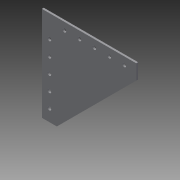
# Autodesk Inventor part: HolonomicCornerBracket
Saved by Autodesk Inventor 2013 SP2 (Build 170200200, 200)
## iProperties
Created: 2015-01-07
Part Number: HolonomicCornerBracket
Material: Generic
Document SubType Name: Sheet Metal
Designer: darkb_000
Density: 1 g/cm^3
Sheet Metal Rule: Default
Author: darkb_000
BendRadius: 0.125 in
BendReliefWidth: 0.125 in
BendReliefDepth: 0.063 in
CornerReliefSize: 0.500 in
MinimumRemnant: 0.250 in
TransitionRadius: 0.125 in
JacobiRadiusSize: 0.125 in
GapSize: 0.125 in
d0: 0.500 in
Thickness: 0.125 in
d1: 0.125 in
d2: 5.000 in
d3: 5.000 in
d4: 1.000 in
d5: 0.125 in
d6: 0.00 deg
d7: 0.125 in
d8: 0.063 in
d9: 0.250 in
d10: 0.125 in
d11: 4.000 in
d12: 90.00 deg
d13: 0.125 in
d14: 0.500 in
d15: 0.125 in
d16: 0.125 in
d17: 0.125 in
d18: 0.00 deg
d19: 1.250 in
d20: 1.250 in
d21: 1.250 in
d22: 1.250 in
d23: 0.125 in
d24: 0.00 deg
Autodesk Inventor part; units mm, degrees
ref_plane "YZ Plane" through (0, 0, 0) normal (1, 0, 0) x (0, 1, 0)
ref_plane "XZ Plane" through (0, 0, 0) normal (0, 1, 0) x (-1, 0, 0)
ref_plane "XY Plane" through (0, 0, 0) normal (0, 0, 1) x (1, 0, 0)
sketch "Sketch1" plane through (0, 0, 0) normal (0, 0, 1) x (1, 0, 0)
  line L0 (-313.0099, -160.8742) -> (-169.3258, -17.1901)
  line L1 (342.9, 12.7) -> (-342.9, 12.7)
  line L2 (-342.9, -12.7) -> (-342.9, -673.1)
  line L3 (-241.1678, -89.0322) -> (-250.1481, -80.0519)
  line L4 (-250.1481, -80.0519) -> (-157.3962, 12.7)
  line L5 (-157.3962, 12.7) -> (-342.9, 12.7)
  line L6 (-157.3962, 12.7) -> (-342.9, -172.8038)
  line L7 (-342.9, -172.8038) -> (-342.9, 12.7)
  circle A0 centre (-203.2, 0) radius 3.175
  circle A1 centre (-228.6, 0) radius 3.175
  circle A2 centre (-254, 0) radius 3.175
  circle A3 centre (-279.4, 0) radius 3.175
  circle A4 centre (-304.8, 0) radius 3.175
  circle A5 centre (-330.2, -25.4) radius 3.175
  circle A6 centre (-330.2, -50.8) radius 3.175
  circle A7 centre (-330.2, -76.2) radius 3.175
  circle A8 centre (-330.2, -101.6) radius 3.175
  circle A9 centre (-330.2, -127) radius 3.175
  line L8 (342.9, -12.7) -> (-342.9, -12.7)
  line L9 (-317.5, -12.7) -> (-317.5, -673.1)
  line L10 (-182.7962, -12.7) -> (-182.7962, 12.7)
  line L11 (-317.5, -147.4038) -> (-342.9, -147.4038)
  point P0 (0, 0)
  dimension "d0" = 12.7
  measures "d0" distance of L3.start L3.end
extrude "Plate1" add sketch "Sketch1" along normal blind 3.175 contours L10 L8 L7 L1 | L4 L6 L9 L8 | L9 L11 L2 L8
sketch "Sketch2" plane through (0, 0, 3.175) normal (0, 0, 1) x (1, 0, 0)
  circle A0 centre (-330.2, -127) radius 3.175 projected
  circle A1 centre (-203.2, 0) radius 3.175 projected
  line L0 (-182.7962, -12.7) -> (-317.5, -147.4038) projected
  line L1 (-342.9, 12.7) -> (-182.7962, 12.7) projected
  line L2 (-342.9, -147.4038) -> (-342.9, 12.7) projected
  line L3 (-317.5, -147.4038) -> (-342.9, -147.4038) projected
  line L4 (-317.5, -114.3) -> (-342.9, -114.3)
  line L5 (-215.9, 12.7) -> (-342.9, 12.7)
  line L6 (-342.9, 12.7) -> (-342.9, -114.3)
  line L7 (-342.9, -114.3) -> (-317.5, -114.3)
  line L8 (-317.5, -114.3) -> (-215.9, -12.7)
  line L9 (-215.9, -114.3) -> (-215.9, -45.8038)
  line L10 (-215.9, -12.7) -> (-215.9, 12.7)
  line L11 (-342.9, -114.3) -> (-317.5, -114.3)
  line L12 (-284.3962, -114.3) -> (-215.9, -114.3)
  line L13 (-215.9, 12.7) -> (-182.7962, 12.7)
  line L14 (-182.7962, 12.7) -> (-182.7962, -12.7)
  line L15 (-182.7962, -12.7) -> (-317.5, -147.4038)
  line L16 (-317.5, -147.4038) -> (-342.9, -147.4038)
  line L17 (-342.9, -147.4038) -> (-342.9, -114.3)
  point P0 (0, 0)
  dimension "d2" = 127
  dimension "d3" = 127
  dimension "d4" = 25.4
  constraints: 28 end point, 6 perpendicular, 5 parallel, 4 collinear, 3 point on line, 2 horizontal
  measures "d2" distance of L5.end L5.start
  measures "d3" distance of L5.start L9.start
  measures "d4" distance of L4.start L4.end
extrude "Cut1" cut sketch "Sketch2" against normal blind 3.175 contours L0 L3 L2 L4 L8 L10 L1 L14
sketch "Sketch3" plane through (-315.2549, -116.5451, -3.175) normal (0.7071068, -0.7071068, 0) x (0.7071068, 0.7071068, 0)
  line L0 (143.6841, 0) -> (0, 0)
  line L1 (0, 0) -> (0, -95.25)
  line L2 (0, -95.25) -> (143.6841, -95.25)
  line L3 (143.6841, -95.25) -> (143.6841, 0)
  constraints: 6 end point, 1 horizontal, 1 perpendicular, 1 vertical
edge flange "Flange1" height 101.6 angle 90 thickness 3.175 bend radius 3.175 thickness toward (0.7071068, -0.7071068, 0) relief tear relief width 3.175 relief depth 1.5875 edges at (-266.7, -63.5, 0) wall of the first edge with corners at (-213.6549, -14.9451, -3.175) (-315.2549, -116.5451, -3.175) (-315.2549, -116.5451, -98.425) (-213.6549, -14.9451, -98.425)
bend "Bend1"
corner "Corner1"
sketch "Sketch4" plane through (-313.0099, -118.7901, -3.175) normal (0.7071068, -0.7071068, 0) x (-0.7071068, -0.7071068, 0)
  line L0 (0, 95.25) -> (0, 0) projected
  line L1 (-174.6104, 73.025) -> (-37.9584, 73.025) projected
  line L2 (-176.1344, 73.025) -> (32.4504, 73.025) projected
  circle A0 centre (-71.842, 34.925) radius 10.8585 projected
  line L3 (0, 73.025) -> (-143.6841, 73.025)
  line L4 (-143.6841, 73.025) -> (-143.6841, 95.25)
  line L5 (-143.6841, 95.25) -> (0, 95.25)
  line L6 (0, 95.25) -> (0, 73.025)
  circle A1 centre (-71.842, 34.925) radius 10.8585
  point P0 (-305.3287, -3.175)
  constraints: 8 end point, 2 parallel, 2 point on line, 1 centre point, 1 coincident, 1 concentric, 1 horizontal, 1 perpendicular
extrude "Cut2" cut sketch "Sketch4" against normal blind 3.175
sketch "Sketch5" plane through (-211.4099, -17.1901, -3.175) normal (0.7071068, -0.7071068, 0) x (-0.7071068, -0.7071068, 0)
  line L0 (0, 73.025) -> (31.75, 73.025)
  line L1 (31.75, 73.025) -> (31.75, 41.275)
  line L2 (31.75, 41.275) -> (0, 41.275)
  line L3 (0, 41.275) -> (0, 73.025)
  line L4 (143.6841, 73.025) -> (111.9341, 73.025)
  line L5 (111.9341, 73.025) -> (111.9341, 41.275)
  line L6 (111.9341, 41.275) -> (143.6841, 41.275)
  line L7 (143.6841, 41.275) -> (143.6841, 73.025)
  line L8 (31.75, 73.025) -> (0, 41.275)
  line L9 (111.9341, 73.025) -> (143.6841, 41.275)
  point P0 (-161.6446, -3.175)
  dimension "d19" = 31.75
  dimension "d20" = 31.75
  dimension "d21" = 31.75
  dimension "d22" = 31.75
  constraints: 20 end point, 4 parallel, 2 horizontal, 2 perpendicular
  measures "d19" distance of L1.end L2.end
  measures "d20" distance of L0.end L1.end
  measures "d21" distance of L6.end L5.end
  measures "d22" distance of L5.end L4.end
extrude "Cut3" cut sketch "Sketch5" against normal blind 3.175 contours L0 L8 L3 | L7 L9 L4
equation "\"d5\" = Thickness"
equation "\"d17\" = Thickness"
equation "\"d23\" = Thickness"
equation "\"d7\" = BendReliefWidth"
equation "\"d8\" = BendReliefDepth"
equation "\"d9\" = MinimumRemnant"
equation "\"d10\" = BendRadius"
equation "\"d13\" = BendRadius"
equation "\"d14\" = CornerReliefSize"
equation "\"d15\" = GapSize"
equation "\"d16\" = JacobiRadiusSize"
equation "\"BendRadius\" = Thickness"
equation "\"BendReliefWidth\" = Thickness"
equation "\"BendReliefDepth\" = 0.5 * Thickness"
equation "\"CornerReliefSize\" = 4 * Thickness"
equation "\"MinimumRemnant\" = 2 * Thickness"
equation "\"TransitionRadius\" = BendRadius"
equation "\"JacobiRadiusSize\" = Thickness"
equation "\"GapSize\" = Thickness"
equation "\"d1\" = BendRadius"
equation "\"Thickness\" = 3.175"
body "Solid1"
